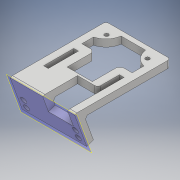
# Autodesk Inventor part: OpenMVMount-Tatev2
Saved by Autodesk Inventor 2018.3 (Build 223284000, 284)
## iProperties
Created: 2019-04-14
Part Number: OpenMVMount-Tatev2
Material: 一般
Document SubType Name: Modeling
Designer: shun2
Density: 1 g/cm^3
Appearance: 既定
Author: shun2
Autodesk Inventor part; units mm, degrees
(part 1 of 6)
ref_plane "YZ Plane" through (0, 0, 0) normal (1, 0, 0) x (0, 1, 0)
ref_plane "XZ Plane" through (0, 0, 0) normal (0, 1, 0) x (-1, 0, 0)
ref_plane "XY Plane" through (0, 0, 0) normal (0, 0, 1) x (1, 0, 0)
sketch "スケッチ1" plane through (0, 0, 0) normal (0, 0, 1) x (1, 0, 0)
  line L0 (0, 44.45) -> (0, 0)
  line L1 (0, 0) -> (35.56, 0)
  line L2 (35.56, 0) -> (35.56, 44.45)
  line L3 (35.56, 44.45) -> (0, 44.45)
  line L4 (3.8608, 3.6322) -> (3.1998, 3.6322)
  line L5 (3.1998, 3.6322) -> (3.1998, 3.9627)
  line L6 (3.1998, 3.9627) -> (3.31, 4.0728)
  line L7 (3.31, 4.0728) -> (3.5303, 4.0728)
  line L8 (3.5303, 4.0728) -> (3.6405, 3.9627)
  line L9 (3.6405, 3.9627) -> (3.6405, 3.6322)
  line L10 (3.1998, 4.8213) -> (3.31, 4.6009)
  line L11 (3.31, 4.6009) -> (3.5303, 4.3806)
  line L12 (3.5303, 4.3806) -> (3.7506, 4.3806)
  line L13 (3.7506, 4.3806) -> (3.8608, 4.4908)
  line L14 (3.8608, 4.4908) -> (3.8608, 4.7111)
  line L15 (3.8608, 4.7111) -> (3.7506, 4.8213)
  line L16 (3.7506, 4.8213) -> (3.6405, 4.8213)
  line L17 (3.6405, 4.8213) -> (3.5303, 4.7111)
  line L18 (3.5303, 4.7111) -> (3.5303, 4.3806)
  line L19 (3.8608, 8.5852) -> (3.1998, 8.5852)
  line L20 (3.1998, 8.5852) -> (3.1998, 8.9157)
  line L21 (3.1998, 8.9157) -> (3.31, 9.0258)
  line L22 (3.31, 9.0258) -> (3.5303, 9.0258)
  line L23 (3.5303, 9.0258) -> (3.6405, 8.9157)
  line L24 (3.6405, 8.9157) -> (3.6405, 8.5852)
  line L25 (3.8608, 9.6641) -> (3.1998, 9.6641)
  line L26 (3.1998, 9.6641) -> (3.5303, 9.3336)
  line L27 (3.5303, 9.3336) -> (3.5303, 9.7743)
  line L28 (3.8608, 6.0452) -> (3.1998, 6.0452)
  line L29 (3.1998, 6.0452) -> (3.1998, 6.3757)
  line L30 (3.1998, 6.3757) -> (3.31, 6.4858)
  line L31 (3.31, 6.4858) -> (3.5303, 6.4858)
  line L32 (3.5303, 6.4858) -> (3.6405, 6.3757)
  line L33 (3.6405, 6.3757) -> (3.6405, 6.0452)
  line L34 (3.1998, 7.2343) -> (3.1998, 6.7936)
  line L35 (3.1998, 6.7936) -> (3.5303, 6.7936)
  line L36 (3.5303, 6.7936) -> (3.4202, 7.0139)
  line L37 (3.4202, 7.0139) -> (3.4202, 7.1241)
  line L38 (3.4202, 7.1241) -> (3.5303, 7.2343)
  line L39 (3.5303, 7.2343) -> (3.7506, 7.2343)
  line L40 (3.7506, 7.2343) -> (3.8608, 7.1241)
  line L41 (3.8608, 7.1241) -> (3.8608, 6.9038)
  line L42 (3.8608, 6.9038) -> (3.7506, 6.7936)
  line L43 (3.8608, 11.1252) -> (3.1998, 11.1252)
  line L44 (3.1998, 11.1252) -> (3.1998, 11.4557)
  line L45 (3.1998, 11.4557) -> (3.31, 11.5658)
  line L46 (3.31, 11.5658) -> (3.5303, 11.5658)
  line L47 (3.5303, 11.5658) -> (3.6405, 11.4557)
  line L48 (3.6405, 11.4557) -> (3.6405, 11.1252)
  line L49 (3.31, 11.8736) -> (3.1998, 11.9838)
  line L50 (3.1998, 11.9838) -> (3.1998, 12.2041)
  line L51 (3.1998, 12.2041) -> (3.31, 12.3143)
  line L52 (3.31, 12.3143) -> (3.4202, 12.3143)
  line L53 (3.4202, 12.3143) -> (3.5303, 12.2041)
  line L54 (3.5303, 12.2041) -> (3.5303, 12.0939)
  line L55 (3.5303, 12.2041) -> (3.6405, 12.3143)
  line L56 (3.6405, 12.3143) -> (3.7506, 12.3143)
  line L57 (3.7506, 12.3143) -> (3.8608, 12.2041)
  line L58 (3.8608, 12.2041) -> (3.8608, 11.9838)
  line L59 (3.8608, 11.9838) -> (3.7506, 11.8736)
  line L60 (3.8608, 13.7922) -> (3.1998, 13.7922)
  line L61 (3.1998, 13.7922) -> (3.1998, 14.1227)
  line L62 (3.1998, 14.1227) -> (3.31, 14.2328)
  line L63 (3.31, 14.2328) -> (3.5303, 14.2328)
  line L64 (3.5303, 14.2328) -> (3.6405, 14.1227)
  line L65 (3.6405, 14.1227) -> (3.6405, 13.7922)
  line L66 (3.8608, 14.9813) -> (3.8608, 14.5406)
  line L67 (3.8608, 14.5406) -> (3.4202, 14.9813)
  line L68 (3.4202, 14.9813) -> (3.31, 14.9813)
  line L69 (3.31, 14.9813) -> (3.1998, 14.8711)
  line L70 (3.1998, 14.8711) -> (3.1998, 14.6508)
  line L71 (3.1998, 14.6508) -> (3.31, 14.5406)
  line L72 (3.8608, 16.3322) -> (3.1998, 16.3322)
  line L73 (3.1998, 16.3322) -> (3.1998, 16.6627)
  line L74 (3.1998, 16.6627) -> (3.31, 16.7728)
  line L75 (3.31, 16.7728) -> (3.5303, 16.7728)
  line L76 (3.5303, 16.7728) -> (3.6405, 16.6627)
  line L77 (3.6405, 16.6627) -> (3.6405, 16.3322)
  line L78 (3.4202, 17.0806) -> (3.1998, 17.3009)
  line L79 (3.1998, 17.3009) -> (3.8608, 17.3009)
  line L80 (3.8608, 17.0806) -> (3.8608, 17.5213)
  line L81 (27.821, 13.7248) -> (27.7108, 13.6147)
  line L82 (27.7108, 13.6147) -> (27.7108, 13.3944)
  line L83 (27.7108, 13.3944) -> (27.821, 13.2842)
  line L84 (27.821, 13.2842) -> (27.9312, 13.2842)
  line L85 (27.9312, 13.2842) -> (28.0413, 13.3944)
  line L86 (28.0413, 13.3944) -> (28.0413, 13.6147)
  line L87 (28.0413, 13.6147) -> (28.1515, 13.7248)
  line L88 (28.1515, 13.7248) -> (28.2616, 13.7248)
  line L89 (28.2616, 13.7248) -> (28.3718, 13.6147)
  line L90 (28.3718, 13.6147) -> (28.3718, 13.3944)
  line L91 (28.3718, 13.3944) -> (28.2616, 13.2842)
  line L92 (27.7108, 14.0326) -> (28.3718, 14.0326)
  line L93 (28.3718, 14.0326) -> (28.1515, 14.2529)
  line L94 (28.1515, 14.2529) -> (28.3718, 14.4733)
  line L95 (28.3718, 14.4733) -> (27.7108, 14.4733)
  line L96 (27.7108, 14.781) -> (28.3718, 14.781)
  line L97 (28.3718, 14.781) -> (28.3718, 15.1115)
  line L98 (28.3718, 15.1115) -> (28.2616, 15.2217)
  line L99 (28.2616, 15.2217) -> (27.821, 15.2217)
  line L100 (27.821, 15.2217) -> (27.7108, 15.1115)
  line L101 (27.7108, 15.1115) -> (27.7108, 14.781)
  line L102 (27.821, 16.2648) -> (27.7108, 16.1547)
  line L103 (27.7108, 16.1547) -> (27.7108, 15.9344)
  line L104 (27.7108, 15.9344) -> (27.821, 15.8242)
  line L105 (27.821, 15.8242) -> (27.9312, 15.8242)
  line L106 (27.9312, 15.8242) -> (28.0413, 15.9344)
  line L107 (28.0413, 15.9344) -> (28.0413, 16.1547)
  line L108 (28.0413, 16.1547) -> (28.1515, 16.2648)
  line L109 (28.1515, 16.2648) -> (28.2616, 16.2648)
  line L110 (28.2616, 16.2648) -> (28.3718, 16.1547)
  line L111 (28.3718, 16.1547) -> (28.3718, 15.9344)
  line L112 (28.3718, 15.9344) -> (28.2616, 15.8242)
  line L113 (27.7108, 16.5726) -> (28.3718, 16.5726)
  line L114 (28.3718, 16.5726) -> (28.1515, 16.7929)
  line L115 (28.1515, 16.7929) -> (28.3718, 17.0133)
  line L116 (28.3718, 17.0133) -> (27.7108, 17.0133)
  line L117 (27.821, 17.7617) -> (27.7108, 17.6515)
  line L118 (27.7108, 17.6515) -> (27.7108, 17.4312)
  line L119 (27.7108, 17.4312) -> (27.821, 17.321)
  line L120 (27.821, 17.321) -> (28.2616, 17.321)
  line L121 (28.2616, 17.321) -> (28.3718, 17.4312)
  line L122 (28.3718, 17.4312) -> (28.3718, 17.6515)
  line L123 (28.3718, 17.6515) -> (28.2616, 17.7617)
  line L124 (32.3088, 15.5067) -> (31.6987, 15.5067)
  line L125 (31.6987, 15.5067) -> (31.6987, 15.8118)
  line L126 (31.6987, 15.8118) -> (31.8004, 15.9134)
  line L127 (31.8004, 15.9134) -> (31.9021, 15.9134)
  line L128 (31.9021, 15.9134) -> (32.0037, 15.8118)
  line L129 (32.0037, 15.8118) -> (32.1054, 15.9134)
  line L130 (32.1054, 15.9134) -> (32.2071, 15.9134)
  line L131 (32.2071, 15.9134) -> (32.3088, 15.8118)
  line L132 (32.3088, 15.8118) -> (32.3088, 15.5067)
  line L133 (32.0037, 15.5067) -> (32.0037, 15.8118)
  line L134 (31.6987, 16.5134) -> (31.6987, 16.31)
  line L135 (31.6987, 16.31) -> (31.8004, 16.2083)
  line L136 (31.8004, 16.2083) -> (32.2071, 16.2083)
  line L137 (32.2071, 16.2083) -> (32.3088, 16.31)
  line L138 (32.3088, 16.31) -> (32.3088, 16.5134)
  line L139 (32.3088, 16.5134) -> (32.2071, 16.6151)
  line L140 (32.2071, 16.6151) -> (31.8004, 16.6151)
  line L141 (31.8004, 16.6151) -> (31.6987, 16.5134)
  line L142 (31.6987, 17.215) -> (31.6987, 17.0117)
  line L143 (31.6987, 17.0117) -> (31.8004, 16.91)
  line L144 (31.8004, 16.91) -> (32.2071, 16.91)
  line L145 (32.2071, 16.91) -> (32.3088, 17.0117)
  line L146 (32.3088, 17.0117) -> (32.3088, 17.215)
  line L147 (32.3088, 17.215) -> (32.2071, 17.3167)
  line L148 (32.2071, 17.3167) -> (31.8004, 17.3167)
  line L149 (31.8004, 17.3167) -> (31.6987, 17.215)
  line L150 (32.3088, 17.815) -> (31.6987, 17.815)
  line L151 (31.6987, 17.6116) -> (31.6987, 18.0184)
  line L152 (32.3088, 18.4912) -> (31.6478, 18.4912)
  line L153 (31.6478, 18.4912) -> (31.6478, 18.8217)
  line L154 (31.6478, 18.8217) -> (31.758, 18.9318)
  line L155 (31.758, 18.9318) -> (31.9783, 18.9318)
  line L156 (31.9783, 18.9318) -> (32.0885, 18.8217)
  line L157 (32.0885, 18.8217) -> (32.0885, 18.4912)
  line L158 (32.0885, 18.7115) -> (32.3088, 18.9318)
  line L159 (31.758, 19.6803) -> (31.6478, 19.5701)
  line L160 (31.6478, 19.5701) -> (31.6478, 19.3498)
  line L161 (31.6478, 19.3498) -> (31.758, 19.2396)
  line L162 (31.758, 19.2396) -> (31.8682, 19.2396)
  line L163 (31.8682, 19.2396) -> (31.9783, 19.3498)
  line L164 (31.9783, 19.3498) -> (31.9783, 19.5701)
  line L165 (31.9783, 19.5701) -> (32.0885, 19.6803)
  line L166 (32.0885, 19.6803) -> (32.1986, 19.6803)
  line L167 (32.1986, 19.6803) -> (32.3088, 19.5701)
  line L168 (32.3088, 19.5701) -> (32.3088, 19.3498)
  line L169 (32.3088, 19.3498) -> (32.1986, 19.2396)
  line L170 (32.3088, 20.2083) -> (31.6478, 20.2083)
  line L171 (31.6478, 19.988) -> (31.6478, 20.4287)
  line L172 (32.3088, 6.1722) -> (31.6478, 6.1722)
  line L173 (31.6478, 6.1722) -> (31.6478, 6.5027)
  line L174 (31.6478, 6.5027) -> (31.758, 6.6128)
  line L175 (31.758, 6.6128) -> (31.9783, 6.6128)
  line L176 (31.9783, 6.6128) -> (32.0885, 6.5027)
  line L177 (32.0885, 6.5027) -> (32.0885, 6.1722)
  line L178 (31.6478, 6.9206) -> (31.6478, 7.3613)
  line L179 (31.6478, 7.3613) -> (31.758, 7.3613)
  line L180 (31.758, 7.3613) -> (32.1986, 6.9206)
  line L181 (32.1986, 6.9206) -> (32.3088, 6.9206)
  line L182 (31.758, 1.1518) -> (31.6478, 1.0417)
  line L183 (31.6478, 1.0417) -> (31.6478, 0.8214)
  line L184 (31.6478, 0.8214) -> (31.758, 0.7112)
  line L185 (31.758, 0.7112) -> (32.1986, 0.7112)
  line L186 (32.1986, 0.7112) -> (32.3088, 0.8214)
  line L187 (32.3088, 0.8214) -> (32.3088, 1.0417)
  line L188 (32.3088, 1.0417) -> (32.1986, 1.1518)
  line L189 (32.1986, 1.1518) -> (31.9783, 1.1518)
  line L190 (31.9783, 1.1518) -> (31.9783, 0.9315)
  line L191 (32.3088, 1.4596) -> (31.6478, 1.4596)
  line L192 (31.6478, 1.4596) -> (32.3088, 1.9003)
  line L193 (32.3088, 1.9003) -> (31.6478, 1.9003)
  line L194 (31.6478, 2.208) -> (32.3088, 2.208)
  line L195 (32.3088, 2.208) -> (32.3088, 2.5385)
  line L196 (32.3088, 2.5385) -> (32.1986, 2.6487)
  line L197 (32.1986, 2.6487) -> (31.758, 2.6487)
  line L198 (31.758, 2.6487) -> (31.6478, 2.5385)
  line L199 (31.6478, 2.5385) -> (31.6478, 2.208)
  line L200 (3.31, 0.5842) -> (3.1998, 0.6944)
  line L201 (3.1998, 0.6944) -> (3.1998, 0.9147)
  line L202 (3.1998, 0.9147) -> (3.31, 1.0248)
  line L203 (3.31, 1.0248) -> (3.4202, 1.0248)
  line L204 (3.4202, 1.0248) -> (3.5303, 0.9147)
  line L205 (3.5303, 0.9147) -> (3.5303, 0.8045)
  line L206 (3.5303, 0.9147) -> (3.6405, 1.0248)
  line L207 (3.6405, 1.0248) -> (3.7506, 1.0248)
  line L208 (3.7506, 1.0248) -> (3.8608, 0.9147)
  line L209 (3.8608, 0.9147) -> (3.8608, 0.6944)
  line L210 (3.8608, 0.6944) -> (3.7506, 0.5842)
  line L211 (3.8608, 1.3326) -> (3.7506, 1.3326)
  line L212 (3.7506, 1.3326) -> (3.7506, 1.4428)
  line L213 (3.7506, 1.4428) -> (3.8608, 1.4428)
  line L214 (3.8608, 1.4428) -> (3.8608, 1.3326)
  line L215 (3.31, 1.7068) -> (3.1998, 1.817)
  line L216 (3.1998, 1.817) -> (3.1998, 2.0373)
  line L217 (3.1998, 2.0373) -> (3.31, 2.1475)
  line L218 (3.31, 2.1475) -> (3.4202, 2.1475)
  line L219 (3.4202, 2.1475) -> (3.5303, 2.0373)
  line L220 (3.5303, 2.0373) -> (3.5303, 1.9271)
  line L221 (3.5303, 2.0373) -> (3.6405, 2.1475)
  line L222 (3.6405, 2.1475) -> (3.7506, 2.1475)
  line L223 (3.7506, 2.1475) -> (3.8608, 2.0373)
  line L224 (3.8608, 2.0373) -> (3.8608, 1.817)
  line L225 (3.8608, 1.817) -> (3.7506, 1.7068)
  line L226 (3.1998, 2.4552) -> (3.6405, 2.4552)
  line L227 (3.6405, 2.4552) -> (3.8608, 2.6756)
  line L228 (3.8608, 2.6756) -> (3.6405, 2.8959)
  line L229 (3.6405, 2.8959) -> (3.1998, 2.8959)
  line L230 (31.6478, 3.2512) -> (32.0885, 3.2512)
  line L231 (32.0885, 3.2512) -> (32.3088, 3.4715)
  line L232 (32.3088, 3.4715) -> (32.0885, 3.6918)
  line L233 (32.0885, 3.6918) -> (31.6478, 3.6918)
  line L234 (32.3088, 3.9996) -> (32.3088, 4.2199)
  line L235 (32.3088, 4.1098) -> (31.6478, 4.1098)
  line L236 (31.6478, 3.9996) -> (31.6478, 4.2199)
  line L237 (32.3088, 4.4986) -> (31.6478, 4.4986)
  line L238 (31.6478, 4.4986) -> (32.3088, 4.9392)
  line L239 (32.3088, 4.9392) -> (31.6478, 4.9392)
  line L240 (32.3088, 8.5852) -> (31.6478, 8.5852)
  line L241 (31.6478, 8.5852) -> (31.6478, 8.9157)
  line L242 (31.6478, 8.9157) -> (31.758, 9.0258)
  line L243 (31.758, 9.0258) -> (31.9783, 9.0258)
  line L244 (31.9783, 9.0258) -> (32.0885, 8.9157)
  line L245 (32.0885, 8.9157) -> (32.0885, 8.5852)
  line L246 (31.758, 9.3336) -> (31.6478, 9.4438)
  line L247 (31.6478, 9.4438) -> (31.6478, 9.6641)
  line L248 (31.6478, 9.6641) -> (31.758, 9.7743)
  line L249 (31.758, 9.7743) -> (31.8682, 9.7743)
  line L250 (31.8682, 9.7743) -> (31.9783, 9.6641)
  line L251 (31.9783, 9.6641) -> (32.0885, 9.7743)
  line L252 (32.0885, 9.7743) -> (32.1986, 9.7743)
  line L253 (32.1986, 9.7743) -> (32.3088, 9.6641)
  line L254 (32.3088, 9.6641) -> (32.3088, 9.4438)
  line L255 (32.3088, 9.4438) -> (32.1986, 9.3336)
  line L256 (32.1986, 9.3336) -> (32.0885, 9.3336)
  line L257 (32.0885, 9.3336) -> (31.9783, 9.4438)
  line L258 (31.9783, 9.4438) -> (31.8682, 9.3336)
  line L259 (31.8682, 9.3336) -> (31.758, 9.3336)
  line L260 (31.9783, 9.4438) -> (31.9783, 9.6641)
  line L261 (3.8608, 18.8722) -> (3.1998, 18.8722)
  line L262 (3.1998, 18.8722) -> (3.1998, 19.2027)
  line L263 (3.1998, 19.2027) -> (3.31, 19.3128)
  line L264 (3.31, 19.3128) -> (3.5303, 19.3128)
  line L265 (3.5303, 19.3128) -> (3.6405, 19.2027)
  line L266 (3.6405, 19.2027) -> (3.6405, 18.8722)
  line L267 (3.7506, 19.6206) -> (3.31, 19.6206)
  line L268 (3.31, 19.6206) -> (3.1998, 19.7308)
  line L269 (3.1998, 19.7308) -> (3.1998, 19.9511)
  line L270 (3.1998, 19.9511) -> (3.31, 20.0613)
  line L271 (3.31, 20.0613) -> (3.7506, 20.0613)
  line L272 (3.7506, 20.0613) -> (3.8608, 19.9511)
  line L273 (3.8608, 19.9511) -> (3.8608, 19.7308)
  line L274 (3.8608, 19.7308) -> (3.7506, 19.6206)
  line L275 (3.7506, 19.6206) -> (3.31, 20.0613)
  line L276 (28.3718, 10.8712) -> (27.7108, 10.8712)
  line L277 (27.7108, 10.8712) -> (27.7108, 11.2017)
  line L278 (27.7108, 11.2017) -> (27.821, 11.3118)
  line L279 (27.821, 11.3118) -> (28.0413, 11.3118)
  line L280 (28.0413, 11.3118) -> (28.1515, 11.2017)
  line L281 (28.1515, 11.2017) -> (28.1515, 10.8712)
  line L282 (28.1515, 11.0915) -> (28.3718, 11.3118)
  line L283 (27.821, 12.0603) -> (27.7108, 11.9501)
  line L284 (27.7108, 11.9501) -> (27.7108, 11.7298)
  line L285 (27.7108, 11.7298) -> (27.821, 11.6196)
  line L286 (27.821, 11.6196) -> (27.9312, 11.6196)
  line L287 (27.9312, 11.6196) -> (28.0413, 11.7298)
  line L288 (28.0413, 11.7298) -> (28.0413, 11.9501)
  line L289 (28.0413, 11.9501) -> (28.1515, 12.0603)
  line L290 (28.1515, 12.0603) -> (28.2616, 12.0603)
  line L291 (28.2616, 12.0603) -> (28.3718, 11.9501)
  line L292 (28.3718, 11.9501) -> (28.3718, 11.7298)
  line L293 (28.3718, 11.7298) -> (28.2616, 11.6196)
  line L294 (28.3718, 12.5884) -> (27.7108, 12.5884)
  line L295 (27.7108, 12.368) -> (27.7108, 12.8087)
  line L296 (27.821, 6.1048) -> (27.7108, 5.9947)
  line L297 (27.7108, 5.9947) -> (27.7108, 5.7744)
  line L298 (27.7108, 5.7744) -> (27.821, 5.6642)
  line L299 (27.821, 5.6642) -> (28.2616, 5.6642)
  line L300 (28.2616, 5.6642) -> (28.3718, 5.7744)
  line L301 (28.3718, 5.7744) -> (28.3718, 5.9947)
  line L302 (28.3718, 5.9947) -> (28.2616, 6.1048)
  line L303 (28.2616, 6.1048) -> (28.0413, 6.1048)
  line L304 (28.0413, 6.1048) -> (28.0413, 5.8845)
  line L305 (28.3718, 6.4126) -> (27.7108, 6.4126)
  line L306 (27.7108, 6.4126) -> (28.3718, 6.8533)
  line L307 (28.3718, 6.8533) -> (27.7108, 6.8533)
  line L308 (27.7108, 7.161) -> (28.3718, 7.161)
  line L309 (28.3718, 7.161) -> (28.3718, 7.4915)
  line L310 (28.3718, 7.4915) -> (28.2616, 7.6017)
  line L311 (28.2616, 7.6017) -> (27.821, 7.6017)
  line L312 (27.821, 7.6017) -> (27.7108, 7.4915)
  line L313 (27.7108, 7.4915) -> (27.7108, 7.161)
  line L314 (27.821, 8.0772) -> (27.7108, 8.1874)
  line L315 (27.7108, 8.1874) -> (27.7108, 8.4077)
  line L316 (27.7108, 8.4077) -> (27.821, 8.5178)
  line L317 (27.821, 8.5178) -> (27.9312, 8.5178)
  line L318 (27.9312, 8.5178) -> (28.0413, 8.4077)
  line L319 (28.0413, 8.4077) -> (28.0413, 8.2975)
  line L320 (28.0413, 8.4077) -> (28.1515, 8.5178)
  line L321 (28.1515, 8.5178) -> (28.2616, 8.5178)
  line L322 (28.2616, 8.5178) -> (28.3718, 8.4077)
  line L323 (28.3718, 8.4077) -> (28.3718, 8.1874)
  line L324 (28.3718, 8.1874) -> (28.2616, 8.0772)
  line L325 (28.3718, 8.8256) -> (28.2616, 8.8256)
  line L326 (28.2616, 8.8256) -> (28.2616, 8.9358)
  line L327 (28.2616, 8.9358) -> (28.3718, 8.9358)
  line L328 (28.3718, 8.9358) -> (28.3718, 8.8256)
  line L329 (27.821, 9.1998) -> (27.7108, 9.31)
  line L330 (27.7108, 9.31) -> (27.7108, 9.5303)
  line L331 (27.7108, 9.5303) -> (27.821, 9.6405)
  line L332 (27.821, 9.6405) -> (27.9312, 9.6405)
  line L333 (27.9312, 9.6405) -> (28.0413, 9.5303)
  line L334 (28.0413, 9.5303) -> (28.0413, 9.4201)
  line L335 (28.0413, 9.5303) -> (28.1515, 9.6405)
  line L336 (28.1515, 9.6405) -> (28.2616, 9.6405)
  line L337 (28.2616, 9.6405) -> (28.3718, 9.5303)
  line L338 (28.3718, 9.5303) -> (28.3718, 9.31)
  line L339 (28.3718, 9.31) -> (28.2616, 9.1998)
  line L340 (27.9312, 9.9482) -> (28.3718, 10.1686)
  line L341 (28.3718, 10.1686) -> (27.9312, 10.3889)
  line L342 (31.758, 13.4708) -> (31.6478, 13.3607)
  line L343 (31.6478, 13.3607) -> (31.6478, 13.1404)
  line L344 (31.6478, 13.1404) -> (31.758, 13.0302)
  line L345 (31.758, 13.0302) -> (31.8682, 13.0302)
  line L346 (31.8682, 13.0302) -> (31.9783, 13.1404)
  line L347 (31.9783, 13.1404) -> (31.9783, 13.3607)
  line L348 (31.9783, 13.3607) -> (32.0885, 13.4708)
  line L349 (32.0885, 13.4708) -> (32.1986, 13.4708)
  line L350 (32.1986, 13.4708) -> (32.3088, 13.3607)
  line L351 (32.3088, 13.3607) -> (32.3088, 13.1404)
  line L352 (32.3088, 13.1404) -> (32.1986, 13.0302)
  line L353 (31.6478, 13.7786) -> (31.758, 13.7786)
  line L354 (31.758, 13.7786) -> (31.9783, 13.9989)
  line L355 (31.9783, 13.9989) -> (31.758, 14.2193)
  line L356 (31.758, 14.2193) -> (31.6478, 14.2193)
  line L357 (31.9783, 13.9989) -> (32.3088, 13.9989)
  line L358 (32.3088, 14.527) -> (31.6478, 14.527)
  line L359 (31.6478, 14.527) -> (32.3088, 14.9677)
  line L360 (32.3088, 14.9677) -> (31.6478, 14.9677)
  line L361 (32.3088, 11.1252) -> (31.6478, 11.1252)
  line L362 (31.6478, 11.1252) -> (31.6478, 11.4557)
  line L363 (31.6478, 11.4557) -> (31.758, 11.5658)
  line L364 (31.758, 11.5658) -> (31.9783, 11.5658)
  line L365 (31.9783, 11.5658) -> (32.0885, 11.4557)
  line L366 (32.0885, 11.4557) -> (32.0885, 11.1252)
  line L367 (32.1986, 11.8736) -> (32.3088, 11.9838)
  line L368 (32.3088, 11.9838) -> (32.3088, 12.2041)
  line L369 (32.3088, 12.2041) -> (32.1986, 12.3143)
  line L370 (32.1986, 12.3143) -> (31.758, 12.3143)
  line L371 (31.758, 12.3143) -> (31.6478, 12.2041)
  line L372 (31.6478, 12.2041) -> (31.6478, 11.9838)
  line L373 (31.6478, 11.9838) -> (31.758, 11.8736)
  line L374 (31.758, 11.8736) -> (31.8682, 11.8736)
  line L375 (31.8682, 11.8736) -> (31.9783, 11.9838)
  line L376 (31.9783, 11.9838) -> (31.9783, 12.3143)
  line L377 (27.878, 25.397) -> (26.478, 25.397)
  line L378 (26.478, 25.397) -> (26.478, 28.197)
  line L379 (26.478, 28.197) -> (27.878, 28.197)
  line L380 (27.878, 28.197) -> (27.878, 25.397)
  line L381 (17.21, 1.902) -> (15.81, 1.902)
  line L382 (15.81, 1.902) -> (15.81, 4.702)
  line L383 (15.81, 4.702) -> (17.21, 4.702)
  line L384 (17.21, 4.702) -> (17.21, 1.902)
  line L385 (7.423, 1.921) -> (7.423, 0.421)
  line L386 (7.423, 0.421) -> (5.023, 0.421)
  line L387 (5.023, 0.421) -> (5.023, 1.921)
  line L388 (7.423, 3.921) -> (7.423, 5.021)
  line L389 (7.423, 5.021) -> (7.023, 5.421)
  line L390 (7.023, 5.421) -> (5.423, 5.421)
  line L391 (5.423, 5.421) -> (5.023, 5.021)
  line L392 (5.023, 5.021) -> (5.023, 3.921)
  line L393 (5.207, 3.302) -> (7.239, 3.302)
  line L394 (8.2855, 10.414) -> (8.2245, 10.414)
  line L395 (8.955, 11.914) -> (8.955, 8.914)
  line L396 (8.955, 8.914) -> (7.555, 8.914)
  line L397 (7.555, 8.914) -> (7.555, 11.914)
  line L398 (7.555, 11.914) -> (8.955, 11.914)
  line L399 (6.6345, 10.414) -> (6.5735, 10.414)
  line L400 (7.304, 11.914) -> (7.304, 8.914)
  line L401 (7.304, 8.914) -> (5.904, 8.914)
  line L402 (5.904, 8.914) -> (5.904, 11.914)
  line L403 (5.904, 11.914) -> (7.304, 11.914)
  line L404 (10.1295, 25.019) -> (10.1905, 25.019)
  line L405 (9.46, 23.519) -> (9.46, 26.519)
  line L406 (9.46, 26.519) -> (10.86, 26.519)
  line L407 (10.86, 26.519) -> (10.86, 23.519)
  line L408 (10.86, 23.519) -> (9.46, 23.519)
  line L409 (12.065, 6.4465) -> (12.065, 6.5075)
  line L410 (13.565, 5.777) -> (10.565, 5.777)
  line L411 (10.565, 5.777) -> (10.565, 7.177)
  line L412 (10.565, 7.177) -> (13.565, 7.177)
  line L413 (13.565, 7.177) -> (13.565, 5.777)
  line L414 (25.5575, 7.747) -> (25.4965, 7.747)
  line L415 (26.227, 9.247) -> (26.227, 6.247)
  line L416 (26.227, 6.247) -> (24.827, 6.247)
  line L417 (24.827, 6.247) -> (24.827, 9.247)
  line L418 (24.827, 9.247) -> (26.227, 9.247)
  line L419 (25.4965, 25.019) -> (25.5575, 25.019)
  line L420 (24.827, 23.519) -> (24.827, 26.519)
  line L421 (24.827, 26.519) -> (26.227, 26.519)
  line L422 (26.227, 26.519) -> (26.227, 23.519)
  line L423 (26.227, 23.519) -> (24.827, 23.519)
  line L424 (28.8595, 26.797) -> (28.7985, 26.797)
  line L425 (29.529, 28.297) -> (29.529, 25.297)
  line L426 (29.529, 25.297) -> (28.129, 25.297)
  line L427 (28.129, 25.297) -> (28.129, 28.297)
  line L428 (28.129, 28.297) -> (29.529, 28.297)
  line L429 (6.928, 26.273) -> (6.928, 27.773)
  line L430 (6.928, 27.773) -> (9.328, 27.773)
  line L431 (9.328, 27.773) -> (9.328, 26.273)
  line L432 (6.928, 24.273) -> (6.928, 23.173)
  line L433 (6.928, 23.173) -> (7.328, 22.773)
  line L434 (7.328, 22.773) -> (8.928, 22.773)
  line L435 (8.928, 22.773) -> (9.328, 23.173)
  line L436 (9.328, 23.173) -> (9.328, 24.273)
  line L437 (9.144, 24.892) -> (7.112, 24.892)
  line L438 (22.971, 41.967) -> (24.471, 41.967)
  line L439 (24.471, 41.967) -> (24.471, 39.567)
  line L440 (24.471, 39.567) -> (22.971, 39.567)
  line L441 (20.971, 41.967) -> (19.871, 41.967)
  line L442 (19.871, 41.967) -> (19.471, 41.567)
  line L443 (19.471, 41.567) -> (19.471, 39.967)
  line L444 (19.471, 39.967) -> (19.871, 39.567)
  line L445 (19.871, 39.567) -> (20.971, 39.567)
  line L446 (21.59, 39.751) -> (21.59, 41.783)
  line L447 (8.2245, 19.812) -> (8.2855, 19.812)
  line L448 (7.555, 18.312) -> (7.555, 21.312)
  line L449 (7.555, 21.312) -> (8.955, 21.312)
  line L450 (8.955, 21.312) -> (8.955, 18.312)
  line L451 (8.955, 18.312) -> (7.555, 18.312)
  line L452 (17.673, 40.4695) -> (17.673, 40.5305)
  line L453 (19.173, 39.8) -> (16.173, 39.8)
  line L454 (16.173, 39.8) -> (16.173, 41.2)
  line L455 (16.173, 41.2) -> (19.173, 41.2)
  line L456 (19.173, 41.2) -> (19.173, 39.8)
  line L457 (22.0305, 35.9) -> (21.9695, 35.9)
  line L458 (22.7, 37.4) -> (22.7, 34.4)
  line L459 (22.7, 34.4) -> (21.3, 34.4)
  line L460 (21.3, 34.4) -> (21.3, 37.4)
  line L461 (21.3, 37.4) -> (22.7, 37.4)
  line L462 (19.3, 32.0695) -> (19.3, 32.1305)
  line L463 (20.8, 31.4) -> (17.8, 31.4)
  line L464 (17.8, 31.4) -> (17.8, 32.8)
  line L465 (17.8, 32.8) -> (20.8, 32.8)
  line L466 (20.8, 32.8) -> (20.8, 31.4)
  line L467 (22.0305, 32.2) -> (21.9695, 32.2)
  line L468 (22.7, 33.7) -> (22.7, 30.7)
  line L469 (22.7, 30.7) -> (21.3, 30.7)
  line L470 (21.3, 30.7) -> (21.3, 33.7)
  line L471 (21.3, 33.7) -> (22.7, 33.7)
  line L472 (13.7305, 37.6) -> (13.6695, 37.6)
  line L473 (14.4, 39.1) -> (14.4, 36.1)
  line L474 (14.4, 36.1) -> (13, 36.1)
  line L475 (13, 36.1) -> (13, 39.1)
  line L476 (13, 39.1) -> (14.4, 39.1)
  line L477 (12.7, 36.2) -> (11.3, 36.2)
  line L478 (11.3, 36.2) -> (11.3, 39)
  line L479 (11.3, 39) -> (12.7, 39)
  line L480 (12.7, 39) -> (12.7, 36.2)
  line L481 (5.842, 14.0005) -> (5.842, 13.9395)
  line L482 (4.342, 14.67) -> (7.342, 14.67)
  line L483 (7.342, 14.67) -> (7.342, 13.27)
  line L484 (7.342, 13.27) -> (4.342, 13.27)
  line L485 (4.342, 13.27) -> (4.342, 14.67)
  line L486 (5.842, 19.5275) -> (5.842, 19.5885)
  line L487 (7.342, 18.858) -> (4.342, 18.858)
  line L488 (4.342, 18.858) -> (4.342, 20.258)
  line L489 (4.342, 20.258) -> (7.342, 20.258)
  line L490 (7.342, 20.258) -> (7.342, 18.858)
  line L491 (29.3586, 19.8336) -> (29.3154, 19.7904)
  line L492 (28.7713, 21.3676) -> (30.8926, 19.2463)
  line L493 (30.8926, 19.2463) -> (29.9027, 18.2564)
  line L494 (29.9027, 18.2564) -> (27.7814, 20.3777)
  line L495 (27.7814, 20.3777) -> (28.7713, 21.3676)
  line L496 (19.685, 6.4465) -> (19.685, 6.5075)
  line L497 (21.185, 5.777) -> (18.185, 5.777)
  line L498 (18.185, 5.777) -> (18.185, 7.177)
  line L499 (18.185, 7.177) -> (21.185, 7.177)
  line L500 (21.185, 7.177) -> (21.185, 5.777)
  line L501 (18.0086, 3.2766) -> (18.0086, 4.0894)
  line L502 (18.0086, 4.0894) -> (18.5674, 4.0894)
  line L503 (20.8534, 4.0894) -> (20.8534, 3.2766)
  line L504 (20.2946, 4.0894) -> (20.8534, 4.0894)
  line L505 (0.381, 41.148) -> (0.635, 41.148)
  line L506 (5.969, 41.148) -> (6.223, 41.148)
  circle A0 centre (3.302, 41.148) radius 2.921
  circle A1 centre (3.302, 41.148) radius 1.5
  line L507 (35.179, 41.148) -> (34.925, 41.148)
  line L508 (29.591, 41.148) -> (29.337, 41.148)
  circle A2 centre (32.258, 41.148) radius 2.921
  circle A3 centre (32.258, 41.148) radius 1.5
  line L509 (35.179, 4.699) -> (35.179, 3.429)
  line L510 (35.179, 3.429) -> (34.544, 2.794)
  line L511 (34.544, 2.794) -> (33.274, 2.794)
  line L512 (33.274, 2.794) -> (32.639, 3.429)
  line L513 (34.544, 7.874) -> (35.179, 7.239)
  line L514 (35.179, 7.239) -> (35.179, 5.969)
  line L515 (35.179, 5.969) -> (34.544, 5.334)
  line L516 (34.544, 5.334) -> (33.274, 5.334)
  line L517 (33.274, 5.334) -> (32.639, 5.969)
  line L518 (32.639, 5.969) -> (32.639, 7.239)
  line L519 (32.639, 7.239) -> (33.274, 7.874)
  line L520 (35.179, 4.699) -> (34.544, 5.334)
  line L521 (33.274, 5.334) -> (32.639, 4.699)
  line L522 (32.639, 3.429) -> (32.639, 4.699)
  line L523 (35.179, 12.319) -> (35.179, 11.049)
  line L524 (35.179, 11.049) -> (34.544, 10.414)
  line L525 (34.544, 10.414) -> (33.274, 10.414)
  line L526 (33.274, 10.414) -> (32.639, 11.049)
  line L527 (34.544, 10.414) -> (35.179, 9.779)
  line L528 (35.179, 9.779) -> (35.179, 8.509)
  line L529 (35.179, 8.509) -> (34.544, 7.874)
  line L530 (34.544, 7.874) -> (33.274, 7.874)
  line L531 (33.274, 7.874) -> (32.639, 8.509)
  line L532 (32.639, 8.509) -> (32.639, 9.779)
  line L533 (32.639, 9.779) -> (33.274, 10.414)
  line L534 (34.544, 15.494) -> (35.179, 14.859)
  line L535 (35.179, 14.859) -> (35.179, 13.589)
  line L536 (35.179, 13.589) -> (34.544, 12.954)
  line L537 (34.544, 12.954) -> (33.274, 12.954)
  line L538 (33.274, 12.954) -> (32.639, 13.589)
  line L539 (32.639, 13.589) -> (32.639, 14.859)
  line L540 (32.639, 14.859) -> (33.274, 15.494)
  line L541 (35.179, 12.319) -> (34.544, 12.954)
  line L542 (33.274, 12.954) -> (32.639, 12.319)
  line L543 (32.639, 11.049) -> (32.639, 12.319)
  line L544 (35.179, 19.939) -> (35.179, 18.669)
  line L545 (35.179, 18.669) -> (34.544, 18.034)
  line L546 (34.544, 18.034) -> (33.274, 18.034)
  line L547 (33.274, 18.034) -> (32.639, 18.669)
  line L548 (34.544, 18.034) -> (35.179, 17.399)
  line L549 (35.179, 17.399) -> (35.179, 16.129)
  line L550 (35.179, 16.129) -> (34.544, 15.494)
  line L551 (34.544, 15.494) -> (33.274, 15.494)
  line L552 (33.274, 15.494) -> (32.639, 16.129)
  line L553 (32.639, 16.129) -> (32.639, 17.399)
  line L554 (32.639, 17.399) -> (33.274, 18.034)
  line L555 (34.544, 20.574) -> (33.274, 20.574)
  line L556 (35.179, 19.939) -> (34.544, 20.574)
  line L557 (33.274, 20.574) -> (32.639, 19.939)
  line L558 (32.639, 18.669) -> (32.639, 19.939)
  line L559 (35.179, 2.159) -> (35.179, 0.889)
  line L560 (35.179, 0.889) -> (34.544, 0.254)
  line L561 (34.544, 0.254) -> (33.274, 0.254)
  line L562 (33.274, 0.254) -> (32.639, 0.889)
  line L563 (35.179, 2.159) -> (34.544, 2.794)
  line L564 (33.274, 2.794) -> (32.639, 2.159)
  line L565 (32.639, 0.889) -> (32.639, 2.159)
  line L566 (2.921, 4.699) -> (2.921, 3.429)
  line L567 (2.921, 3.429) -> (2.286, 2.794)
  line L568 (2.286, 2.794) -> (1.016, 2.794)
  line L569 (1.016, 2.794) -> (0.381, 3.429)
  line L570 (2.286, 7.874) -> (2.921, 7.239)
  line L571 (2.921, 7.239) -> (2.921, 5.969)
  line L572 (2.921, 5.969) -> (2.286, 5.334)
  line L573 (2.286, 5.334) -> (1.016, 5.334)
  line L574 (1.016, 5.334) -> (0.381, 5.969)
  line L575 (0.381, 5.969) -> (0.381, 7.239)
  line L576 (0.381, 7.239) -> (1.016, 7.874)
  line L577 (2.921, 4.699) -> (2.286, 5.334)
  line L578 (1.016, 5.334) -> (0.381, 4.699)
  line L579 (0.381, 3.429) -> (0.381, 4.699)
  line L580 (2.921, 12.319) -> (2.921, 11.049)
  line L581 (2.921, 11.049) -> (2.286, 10.414)
  line L582 (2.286, 10.414) -> (1.016, 10.414)
  line L583 (1.016, 10.414) -> (0.381, 11.049)
  line L584 (2.286, 10.414) -> (2.921, 9.779)
  line L585 (2.921, 9.779) -> (2.921, 8.509)
  line L586 (2.921, 8.509) -> (2.286, 7.874)
  line L587 (2.286, 7.874) -> (1.016, 7.874)
  line L588 (1.016, 7.874) -> (0.381, 8.509)
  line L589 (0.381, 8.509) -> (0.381, 9.779)
  line L590 (0.381, 9.779) -> (1.016, 10.414)
  line L591 (2.286, 15.494) -> (2.921, 14.859)
  line L592 (2.921, 14.859) -> (2.921, 13.589)
  line L593 (2.921, 13.589) -> (2.286, 12.954)
  line L594 (2.286, 12.954) -> (1.016, 12.954)
  line L595 (1.016, 12.954) -> (0.381, 13.589)
  line L596 (0.381, 13.589) -> (0.381, 14.859)
  line L597 (0.381, 14.859) -> (1.016, 15.494)
  line L598 (2.921, 12.319) -> (2.286, 12.954)
  line L599 (1.016, 12.954) -> (0.381, 12.319)
  line L600 (0.381, 11.049) -> (0.381, 12.319)
  line L601 (2.921, 19.939) -> (2.921, 18.669)
  line L602 (2.921, 18.669) -> (2.286, 18.034)
  line L603 (2.286, 18.034) -> (1.016, 18.034)
  line L604 (1.016, 18.034) -> (0.381, 18.669)
  line L605 (2.286, 18.034) -> (2.921, 17.399)
  line L606 (2.921, 17.399) -> (2.921, 16.129)
  line L607 (2.921, 16.129) -> (2.286, 15.494)
  line L608 (2.286, 15.494) -> (1.016, 15.494)
  line L609 (1.016, 15.494) -> (0.381, 16.129)
  line L610 (0.381, 16.129) -> (0.381, 17.399)
  line L611 (0.381, 17.399) -> (1.016, 18.034)
  line L612 (2.286, 20.574) -> (1.016, 20.574)
  line L613 (2.921, 19.939) -> (2.286, 20.574)
  line L614 (1.016, 20.574) -> (0.381, 19.939)
  line L615 (0.381, 18.669) -> (0.381, 19.939)
  line L616 (2.921, 2.159) -> (2.921, 0.889)
  line L617 (2.921, 0.889) -> (2.286, 0.254)
  line L618 (2.286, 0.254) -> (1.016, 0.254)
  line L619 (1.016, 0.254) -> (0.381, 0.889)
  line L620 (2.921, 2.159) -> (2.286, 2.794)
  line L621 (1.016, 2.794) -> (0.381, 2.159)
  line L622 (0.381, 0.889) -> (0.381, 2.159)
  line L623 (31.369, 9.779) -> (31.369, 8.509)
  line L624 (31.369, 8.509) -> (30.734, 7.874)
  line L625 (30.734, 7.874) -> (29.464, 7.874)
  line L626 (29.464, 7.874) -> (28.829, 8.509)
  line L627 (30.734, 12.954) -> (31.369, 12.319)
  line L628 (31.369, 12.319) -> (31.369, 11.049)
  line L629 (31.369, 11.049) -> (30.734, 10.414)
  line L630 (30.734, 10.414) -> (29.464, 10.414)
  line L631 (29.464, 10.414) -> (28.829, 11.049)
  line L632 (28.829, 11.049) -> (28.829, 12.319)
  line L633 (28.829, 12.319) -> (29.464, 12.954)
  line L634 (31.369, 9.779) -> (30.734, 10.414)
  line L635 (29.464, 10.414) -> (28.829, 9.779)
  line L636 (28.829, 8.509) -> (28.829, 9.779)
  line L637 (31.369, 17.399) -> (31.369, 16.129)
  line L638 (31.369, 16.129) -> (30.734, 15.494)
  line L639 (30.734, 15.494) -> (29.464, 15.494)
  line L640 (29.464, 15.494) -> (28.829, 16.129)
  line L641 (30.734, 15.494) -> (31.369, 14.859)
  line L642 (31.369, 14.859) -> (31.369, 13.589)
  line L643 (31.369, 13.589) -> (30.734, 12.954)
  line L644 (30.734, 12.954) -> (29.464, 12.954)
  line L645 (29.464, 12.954) -> (28.829, 13.589)
  line L646 (28.829, 13.589) -> (28.829, 14.859)
  line L647 (28.829, 14.859) -> (29.464, 15.494)
  line L648 (30.734, 18.034) -> (29.464, 18.034)
  line L649 (31.369, 17.399) -> (30.734, 18.034)
  line L650 (29.464, 18.034) -> (28.829, 17.399)
  line L651 (28.829, 16.129) -> (28.829, 17.399)
  line L652 (31.369, 7.239) -> (31.369, 5.969)
  line L653 (31.369, 5.969) -> (30.734, 5.334)
  line L654 (30.734, 5.334) -> (29.464, 5.334)
  line L655 (29.464, 5.334) -> (28.829, 5.969)
  line L656 (31.369, 7.239) -> (30.734, 7.874)
  line L657 (29.464, 7.874) -> (28.829, 7.239)
  line L658 (28.829, 5.969) -> (28.829, 7.239)
  line L659 (5.653, 11.914) -> (5.653, 8.914)
  line L660 (5.653, 8.914) -> (4.253, 8.914)
  line L661 (4.253, 8.914) -> (4.253, 11.914)
  line L662 (4.253, 11.914) -> (5.653, 11.914)
  line L663 (24.487, 5.777) -> (21.487, 5.777)
  line L664 (21.487, 5.777) -> (21.487, 7.177)
  line L665 (21.487, 7.177) -> (24.487, 7.177)
  line L666 (24.487, 7.177) -> (24.487, 5.777)
  line L667 (1.24, 31.399) -> (0.94, 31.399)
  line L668 (0.94, 31.399) -> (0.94, 28.799)
  line L669 (0.94, 28.799) -> (1.24, 28.799)
  line L670 (3.84, 31.399) -> (4.14, 31.399)
  line L671 (4.14, 31.399) -> (4.14, 28.799)
  line L672 (4.14, 28.799) -> (3.84, 28.799)
  line L673 (3.94, 31.899) -> (3.94, 32.499)
  line L674 (3.94, 32.499) -> (3.34, 32.499)
  line L675 (33.1614, 34.4142) -> (33.5857, 33.9899)
  line L676 (33.5857, 33.9899) -> (34.7171, 35.1213)
  line L677 (34.7171, 35.1213) -> (34.2928, 35.5456)
  line L678 (31.7472, 35.8284) -> (31.3229, 36.2527)
  line L679 (31.3229, 36.2527) -> (32.4543, 37.3841)
  line L680 (32.4543, 37.3841) -> (32.8786, 36.9598)
  line L681 (32.3129, 35.4042) -> (32.8079, 35.8991)
  line L682 (32.8079, 35.8991) -> (33.3028, 36.3941)
  line L683 (32.8079, 35.8991) -> (32.8079, 35.0506)
  line L684 (32.8079, 35.0506) -> (33.6564, 35.8991)
  line L685 (33.6564, 35.8991) -> (32.8079, 35.8991)
  line L686 (3.8128, 35.8284) -> (4.2371, 36.2527)
  line L687 (4.2371, 36.2527) -> (3.1057, 37.3841)
  line L688 (3.1057, 37.3841) -> (2.6814, 36.9598)
  line L689 (2.3986, 34.4142) -> (1.9743, 33.9899)
  line L690 (1.9743, 33.9899) -> (0.8429, 35.1213)
  line L691 (0.8429, 35.1213) -> (1.2672, 35.5456)
  line L692 (2.8228, 34.9799) -> (2.3279, 35.4749)
  line L693 (2.3279, 35.4749) -> (1.8329, 35.9698)
  line L694 (2.3279, 35.4749) -> (3.1764, 35.4749)
  line L695 (3.1764, 35.4749) -> (2.3279, 36.3234)
  line L696 (2.3279, 36.3234) -> (2.3279, 35.4749)
  line L697 (9.78, 28.068) -> (9.78, 34.091)
  line L698 (9.78, 34.091) -> (9.78, 38.045)
  line L699 (9.78, 38.045) -> (9.78, 44.068)
  line L700 (9.78, 44.068) -> (25.78, 44.068)
  line L701 (25.78, 44.068) -> (25.78, 38.045)
  line L702 (25.78, 38.045) -> (25.78, 34.091)
  line L703 (25.78, 34.091) -> (25.78, 28.068)
  line L704 (25.78, 28.068) -> (9.78, 28.068)
  arc A4 (9.78, 38.045) -> (9.78, 34.091) centre (7.803, 36.068) ccw
  arc A5 (25.78, 34.091) -> (25.78, 38.045) centre (27.757, 36.068) ccw
  line L705 (10.78, 29.068) -> (24.78, 29.068)
  line L706 (24.78, 29.068) -> (24.78, 43.068)
  line L707 (24.78, 43.068) -> (10.78, 43.068)
  line L708 (10.78, 43.068) -> (10.78, 29.068)
  line L709 (27.051, 40.005) -> (26.67, 39.878)
  line L710 (26.67, 39.878) -> (26.543, 40.005)
  line L711 (26.543, 40.005) -> (26.797, 40.386)
  line L712 (26.797, 40.386) -> (26.543, 40.767)
  line L713 (26.543, 40.767) -> (26.289, 40.767)
  line L714 (26.289, 40.767) -> (26.289, 41.021)
  line L715 (26.289, 41.021) -> (26.67, 41.021)
  line L716 (26.67, 41.021) -> (26.797, 41.402)
  line L717 (26.797, 41.402) -> (26.543, 41.783)
  line L718 (26.543, 41.783) -> (26.67, 41.91)
  line L719 (26.67, 41.91) -> (27.051, 41.656)
  line L720 (27.051, 41.656) -> (27.432, 41.91)
  line L721 (27.432, 41.91) -> (27.432, 42.164)
  line L722 (27.432, 42.164) -> (27.686, 42.164)
  line L723 (27.686, 42.164) -> (27.813, 41.783)
  line L724 (27.813, 41.783) -> (28.194, 41.656)
  line L725 (28.194, 41.656) -> (28.448, 41.91)
  line L726 (28.448, 41.91) -> (28.575, 41.783)
  line L727 (28.575, 41.783) -> (28.448, 41.402)
  line L728 (28.448, 41.402) -> (28.575, 41.021)
  line L729 (28.575, 41.021) -> (28.956, 41.021)
  line L730 (28.956, 41.021) -> (28.829, 40.767)
  line L731 (28.829, 40.767) -> (28.448, 40.64)
  line L732 (28.448, 40.64) -> (28.448, 40.259)
  line L733 (28.448, 40.259) -> (28.575, 40.005)
  line L734 (28.575, 40.005) -> (28.448, 39.878)
  line L735 (28.448, 39.878) -> (28.194, 40.005)
  line L736 (28.194, 40.005) -> (28.067, 40.005)
  line L737 (28.067, 40.005) -> (27.94, 40.386)
  line L738 (27.94, 40.386) -> (28.194, 40.894)
  line L739 (28.194, 40.894) -> (27.94, 41.275)
  line L740 (27.94, 41.275) -> (27.559, 41.402)
  line L741 (27.559, 41.402) -> (27.178, 41.275)
  line L742 (27.178, 41.275) -> (27.051, 40.894)
  line L743 (27.051, 40.894) -> (27.178, 40.513)
  line L744 (27.178, 40.513) -> (27.305, 40.386)
  line L745 (27.305, 40.386) -> (27.051, 40.005)
  line L746 (26.6192, 39.9288) -> (26.8224, 39.9288)
  line L747 (28.3464, 39.9288) -> (28.4988, 39.9288)
  line L748 (26.5938, 40.0812) -> (27.1018, 40.0812)
  line L749 (28.0416, 40.0812) -> (28.5369, 40.0812)
  line L750 (26.6954, 40.2336) -> (27.2034, 40.2336)
  line L751 (27.9908, 40.2336) -> (28.4607, 40.2336)
  line L752 (26.797, 40.386) -> (27.305, 40.386)
  line L753 (27.94, 40.386) -> (28.448, 40.386)
  line L754 (26.6954, 40.5384) -> (27.1695, 40.5384)
  line L755 (28.0162, 40.5384) -> (28.448, 40.5384)
  line L756 (26.5938, 40.6908) -> (27.1187, 40.6908)
  line L757 (28.0924, 40.6908) -> (28.6004, 40.6908)
  line L758 (26.289, 40.8432) -> (27.0679, 40.8432)
  line L759 (28.1686, 40.8432) -> (28.8671, 40.8432)
  line L760 (26.289, 40.9956) -> (27.0849, 40.9956)
  line L761 (28.1263, 40.9956) -> (28.9433, 40.9956)
  line L762 (26.7123, 41.148) -> (27.1357, 41.148)
  line L763 (28.0247, 41.148) -> (28.5327, 41.148)
  line L764 (26.7631, 41.3004) -> (27.2542, 41.3004)
  line L765 (27.8638, 41.3004) -> (28.4819, 41.3004)
  line L766 (26.7631, 41.4528) -> (28.4649, 41.4528)
  line L767 (26.6615, 41.6052) -> (28.5157, 41.6052)
  line L768 (26.5599, 41.7576) -> (26.8986, 41.7576)
  line L769 (27.2034, 41.7576) -> (27.8892, 41.7576)
  line L770 (28.2956, 41.7576) -> (28.5665, 41.7576)
  line L771 (27.432, 41.91) -> (27.7707, 41.91)
  line L772 (27.432, 42.0624) -> (27.7199, 42.0624)
  line L773 (27.3812, 40.4622) -> (27.1272, 39.878)
  line L774 (27.1272, 39.878) -> (27.0002, 39.9542)
  line L775 (27.0002, 39.9542) -> (26.6954, 39.751)
  line L776 (26.6954, 39.751) -> (26.4668, 39.9796)
  line L777 (26.4668, 39.9796) -> (26.67, 40.3098)
  line L778 (26.67, 40.3098) -> (26.543, 40.64)
  line L779 (26.543, 40.64) -> (26.162, 40.7162)
  line L780 (26.162, 40.7162) -> (26.162, 41.0464)
  line L781 (26.162, 41.0464) -> (26.543, 41.0972)
  line L782 (26.543, 41.0972) -> (26.6954, 41.4274)
  line L783 (26.6954, 41.4274) -> (26.4668, 41.7576)
  line L784 (26.4668, 41.7576) -> (26.6954, 41.9862)
  line L785 (26.6954, 41.9862) -> (27.0256, 41.7576)
  line L786 (27.0256, 41.7576) -> (27.3304, 41.8846)
  line L787 (27.3304, 41.8846) -> (27.4066, 42.291)
  line L788 (27.4066, 42.291) -> (27.7368, 42.291)
  line L789 (27.7368, 42.291) -> (27.813, 41.8846)
  line L790 (27.813, 41.8846) -> (28.1178, 41.7576)
  line L791 (28.1178, 41.7576) -> (28.4734, 41.9862)
  line L792 (28.4734, 41.9862) -> (28.702, 41.7576)
  line L793 (28.702, 41.7576) -> (28.4734, 41.4274)
  line L794 (28.4734, 41.4274) -> (28.6004, 41.1226)
  line L795 (28.6004, 41.1226) -> (28.9814, 41.0464)
  line L796 (28.9814, 41.0464) -> (28.9814, 40.7162)
  line L797 (28.9814, 40.7162) -> (28.6258, 40.64)
  line L798 (28.6258, 40.64) -> (28.4734, 40.3098)
  line L799 (28.4734, 40.3098) -> (28.702, 39.9796)
  line L800 (28.702, 39.9796) -> (28.4734, 39.751)
  line L801 (28.4734, 39.751) -> (28.1686, 39.9542)
  line L802 (28.1686, 39.9542) -> (28.0162, 39.878)
  line L803 (28.0162, 39.878) -> (27.7876, 40.4622)
  arc A6 (27.7876, 40.4622) -> (27.3812, 40.4622) centre (27.5844, 40.8686) ccw
  line L804 (2.756, 25.719) -> (2.156, 25.719)
  line L805 (2.156, 25.719) -> (2.156, 24.919)
  line L806 (4.356, 25.719) -> (4.956, 25.719)
  line L807 (4.956, 25.719) -> (4.956, 24.919)
  line L808 (6.669, 26.519) -> (6.669, 23.519)
  line L809 (6.669, 23.519) -> (5.269, 23.519)
  line L810 (5.269, 23.519) -> (5.269, 26.519)
  line L811 (5.269, 26.519) -> (6.669, 26.519)
  line L812 (1.843, 26.519) -> (1.843, 23.519)
  line L813 (1.843, 23.519) -> (0.443, 23.519)
  line L814 (0.443, 23.519) -> (0.443, 26.519)
  line L815 (0.443, 26.519) -> (1.843, 26.519)
  line L816 (20.804, 29.399) -> (17.804, 29.399)
  line L817 (17.804, 29.399) -> (17.804, 30.799)
  line L818 (17.804, 30.799) -> (20.804, 30.799)
  line L819 (20.804, 30.799) -> (20.804, 29.399)
  line L820 (24.4, 33.7) -> (24.4, 30.7)
  line L821 (24.4, 30.7) -> (23, 30.7)
  line L822 (23, 30.7) -> (23, 33.7)
  line L823 (23, 33.7) -> (24.4, 33.7)
  line L824 (7.1635, 28.803) -> (5.6635, 28.803)
  line L825 (5.6635, 31.903) -> (7.1635, 31.903)
  line L826 (28.817, 21.691) -> (27.317, 21.691)
  line L827 (27.317, 24.791) -> (28.817, 24.791)
  line L828 (28.817, 29.184) -> (27.317, 29.184)
  line L829 (27.317, 32.284) -> (28.817, 32.284)
  line L830 (15.35, 32.35) -> (15.35, 30.85)
  line L831 (13.85, 30.85) -> (13.85, 32.35)
  line L832 (11.38, 9.483) -> (24.18, 9.483)
  line L833 (24.68, 9.983) -> (24.68, 22.783)
  line L834 (24.18, 23.283) -> (11.38, 23.283)
  line L835 (11.38, 23.283) -> (10.88, 22.783)
  line L836 (10.88, 22.783) -> (10.88, 9.983)
  line L837 (24.18, 23.283) -> (24.68, 22.783)
  line L838 (24.18, 9.483) -> (24.68, 9.983)
  line L839 (11.38, 9.483) -> (10.88, 9.983)
  circle A7 centre (11.88, 22.283) radius 0.5
  line L840 (20.575, 33.775) -> (15.225, 33.775)
  line L841 (15.225, 33.775) -> (15.225, 39.025)
  line L842 (15.225, 39.025) -> (20.575, 39.025)
  line L843 (20.575, 39.025) -> (20.575, 33.775)
  line L844 (13.203, 0.394) -> (9.403, 0.394)
  line L845 (9.403, 0.394) -> (9.403, 5.194)
  line L846 (9.403, 5.194) -> (13.203, 5.194)
  line L847 (13.203, 5.194) -> (13.203, 0.394)
  circle A8 centre (9.903, 4.694) radius 0.15
  line L848 (35.466, 20.943) -> (35.466, 32.943)
  line L849 (35.466, 32.943) -> (29.866, 32.943)
  line L850 (29.866, 32.943) -> (29.866, 20.943)
  line L851 (29.866, 20.943) -> (35.466, 20.943)
  line L852 (22.09, 0.0025) -> (31.25, 0.0025)
  line L853 (22.09, 0.0025) -> (22.09, 5.1575)
  line L854 (22.09, 5.1575) -> (31.25, 5.1575)
  line L855 (31.25, 5.1575) -> (31.25, 0.0025)
  line L856 (7.388, 17.402) -> (7.388, 16.202)
  line L857 (6.238, 15.152) -> (5.638, 15.152)
  line L858 (4.488, 16.202) -> (4.488, 17.402)
  line L859 (6.288, 18.402) -> (5.688, 18.402)
  circle A9 centre (4.519, 18.414) radius 0.1
  line L860 (26.678, 28.197) -> (26.678, 27.197)
  line L861 (26.678, 27.197) -> (27.678, 27.197)
  line L862 (27.678, 27.197) -> (27.678, 28.197)
  line L863 (27.678, 28.197) -> (26.678, 28.197)
  line L864 (26.678, 26.397) -> (26.678, 25.397)
  line L865 (26.678, 25.397) -> (27.678, 25.397)
  line L866 (27.678, 25.397) -> (27.678, 26.397)
  line L867 (27.678, 26.397) -> (26.678, 26.397)
  line L868 (16.01, 4.702) -> (16.01, 3.702)
  line L869 (16.01, 3.702) -> (17.01, 3.702)
  line L870 (17.01, 3.702) -> (17.01, 4.702)
  line L871 (17.01, 4.702) -> (16.01, 4.702)
  line L872 (16.01, 2.902) -> (16.01, 1.902)
  line L873 (16.01, 1.902) -> (17.01, 1.902)
  line L874 (17.01, 1.902) -> (17.01, 2.902)
  line L875 (17.01, 2.902) -> (16.01, 2.902)
  line L876 (6.723, 4.821) -> (5.723, 4.821)
  line L877 (5.723, 4.821) -> (5.723, 3.821)
  line L878 (5.723, 3.821) -> (6.723, 3.821)
  line L879 (6.723, 3.821) -> (6.723, 4.821)
  line L880 (6.723, 2.021) -> (5.723, 2.021)
  line L881 (5.723, 2.021) -> (5.723, 1.021)
  line L882 (5.723, 1.021) -> (6.723, 1.021)
  line L883 (6.723, 1.021) -> (6.723, 2.021)
  line L884 (7.755, 11.714) -> (7.755, 10.714)
  line L885 (7.755, 10.714) -> (8.755, 10.714)
  line L886 (8.755, 10.714) -> (8.755, 11.714)
  line L887 (8.755, 11.714) -> (7.755, 11.714)
  line L888 (7.755, 10.114) -> (7.755, 9.114)
  line L889 (7.755, 9.114) -> (8.755, 9.114)
  line L890 (8.755, 9.114) -> (8.755, 10.114)
  line L891 (8.755, 10.114) -> (7.755, 10.114)
  line L892 (6.104, 11.714) -> (6.104, 10.714)
  line L893 (6.104, 10.714) -> (7.104, 10.714)
  line L894 (7.104, 10.714) -> (7.104, 11.714)
  line L895 (7.104, 11.714) -> (6.104, 11.714)
  line L896 (6.104, 10.114) -> (6.104, 9.114)
  line L897 (6.104, 9.114) -> (7.104, 9.114)
  line L898 (7.104, 9.114) -> (7.104, 10.114)
  line L899 (7.104, 10.114) -> (6.104, 10.114)
  line L900 (10.66, 23.719) -> (10.66, 24.719)
  line L901 (10.66, 24.719) -> (9.66, 24.719)
  line L902 (9.66, 24.719) -> (9.66, 23.719)
  line L903 (9.66, 23.719) -> (10.66, 23.719)
  line L904 (10.66, 25.319) -> (10.66, 26.319)
  line L905 (10.66, 26.319) -> (9.66, 26.319)
  line L906 (9.66, 26.319) -> (9.66, 25.319)
  line L907 (9.66, 25.319) -> (10.66, 25.319)
  line L908 (13.365, 6.977) -> (12.365, 6.977)
  line L909 (12.365, 6.977) -> (12.365, 5.977)
  line L910 (12.365, 5.977) -> (13.365, 5.977)
  line L911 (13.365, 5.977) -> (13.365, 6.977)
  line L912 (11.765, 6.977) -> (10.765, 6.977)
  line L913 (10.765, 6.977) -> (10.765, 5.977)
  line L914 (10.765, 5.977) -> (11.765, 5.977)
  line L915 (11.765, 5.977) -> (11.765, 6.977)
  line L916 (25.027, 9.047) -> (25.027, 8.047)
  line L917 (25.027, 8.047) -> (26.027, 8.047)
  line L918 (26.027, 8.047) -> (26.027, 9.047)
  line L919 (26.027, 9.047) -> (25.027, 9.047)
  line L920 (25.027, 7.447) -> (25.027, 6.447)
  line L921 (25.027, 6.447) -> (26.027, 6.447)
  line L922 (26.027, 6.447) -> (26.027, 7.447)
  line L923 (26.027, 7.447) -> (25.027, 7.447)
  line L924 (26.027, 23.719) -> (26.027, 24.719)
  line L925 (26.027, 24.719) -> (25.027, 24.719)
  line L926 (25.027, 24.719) -> (25.027, 23.719)
  line L927 (25.027, 23.719) -> (26.027, 23.719)
  line L928 (26.027, 25.319) -> (26.027, 26.319)
  line L929 (26.027, 26.319) -> (25.027, 26.319)
  line L930 (25.027, 26.319) -> (25.027, 25.319)
  line L931 (25.027, 25.319) -> (26.027, 25.319)
  line L932 (28.329, 28.097) -> (28.329, 27.097)
  line L933 (28.329, 27.097) -> (29.329, 27.097)
  line L934 (29.329, 27.097) -> (29.329, 28.097)
  line L935 (29.329, 28.097) -> (28.329, 28.097)
  line L936 (28.329, 26.497) -> (28.329, 25.497)
  line L937 (28.329, 25.497) -> (29.329, 25.497)
  line L938 (29.329, 25.497) -> (29.329, 26.497)
  line L939 (29.329, 26.497) -> (28.329, 26.497)
  line L940 (7.628, 23.373) -> (8.628, 23.373)
  line L941 (8.628, 23.373) -> (8.628, 24.373)
  line L942 (8.628, 24.373) -> (7.628, 24.373)
  line L943 (7.628, 24.373) -> (7.628, 23.373)
  line L944 (7.628, 26.173) -> (8.628, 26.173)
  line L945 (8.628, 26.173) -> (8.628, 27.173)
  line L946 (8.628, 27.173) -> (7.628, 27.173)
  line L947 (7.628, 27.173) -> (7.628, 26.173)
  line L948 (20.071, 41.267) -> (20.071, 40.267)
  line L949 (20.071, 40.267) -> (21.071, 40.267)
  line L950 (21.071, 40.267) -> (21.071, 41.267)
  line L951 (21.071, 41.267) -> (20.071, 41.267)
  line L952 (22.871, 41.267) -> (22.871, 40.267)
  line L953 (22.871, 40.267) -> (23.871, 40.267)
  line L954 (23.871, 40.267) -> (23.871, 41.267)
  line L955 (23.871, 41.267) -> (22.871, 41.267)
  line L956 (8.755, 18.512) -> (8.755, 19.512)
  line L957 (8.755, 19.512) -> (7.755, 19.512)
  line L958 (7.755, 19.512) -> (7.755, 18.512)
  line L959 (7.755, 18.512) -> (8.755, 18.512)
  line L960 (8.755, 20.112) -> (8.755, 21.112)
  line L961 (8.755, 21.112) -> (7.755, 21.112)
  line L962 (7.755, 21.112) -> (7.755, 20.112)
  line L963 (7.755, 20.112) -> (8.755, 20.112)
  line L964 (18.973, 41) -> (17.973, 41)
  line L965 (17.973, 41) -> (17.973, 40)
  line L966 (17.973, 40) -> (18.973, 40)
  line L967 (18.973, 40) -> (18.973, 41)
  line L968 (17.373, 41) -> (16.373, 41)
  line L969 (16.373, 41) -> (16.373, 40)
  line L970 (16.373, 40) -> (17.373, 40)
  line L971 (17.373, 40) -> (17.373, 41)
  line L972 (21.5, 37.2) -> (21.5, 36.2)
  line L973 (21.5, 36.2) -> (22.5, 36.2)
  line L974 (22.5, 36.2) -> (22.5, 37.2)
  line L975 (22.5, 37.2) -> (21.5, 37.2)
  line L976 (21.5, 35.6) -> (21.5, 34.6)
  line L977 (21.5, 34.6) -> (22.5, 34.6)
  line L978 (22.5, 34.6) -> (22.5, 35.6)
  line L979 (22.5, 35.6) -> (21.5, 35.6)
  line L980 (20.6, 32.6) -> (19.6, 32.6)
  line L981 (19.6, 32.6) -> (19.6, 31.6)
  line L982 (19.6, 31.6) -> (20.6, 31.6)
  line L983 (20.6, 31.6) -> (20.6, 32.6)
  line L984 (19, 32.6) -> (18, 32.6)
  line L985 (18, 32.6) -> (18, 31.6)
  line L986 (18, 31.6) -> (19, 31.6)
  line L987 (19, 31.6) -> (19, 32.6)
  line L988 (21.5, 33.5) -> (21.5, 32.5)
  line L989 (21.5, 32.5) -> (22.5, 32.5)
  line L990 (22.5, 32.5) -> (22.5, 33.5)
  line L991 (22.5, 33.5) -> (21.5, 33.5)
  line L992 (21.5, 31.9) -> (21.5, 30.9)
  line L993 (21.5, 30.9) -> (22.5, 30.9)
  line L994 (22.5, 30.9) -> (22.5, 31.9)
  line L995 (22.5, 31.9) -> (21.5, 31.9)
  line L996 (13.2, 38.9) -> (13.2, 37.9)
  line L997 (13.2, 37.9) -> (14.2, 37.9)
  line L998 (14.2, 37.9) -> (14.2, 38.9)
  line L999 (14.2, 38.9) -> (13.2, 38.9)
  line L1000 (13.2, 37.3) -> (13.2, 36.3)
  line L1001 (13.2, 36.3) -> (14.2, 36.3)
  line L1002 (14.2, 36.3) -> (14.2, 37.3)
  line L1003 (14.2, 37.3) -> (13.2, 37.3)
  line L1004 (11.5, 39) -> (11.5, 38)
  line L1005 (11.5, 38) -> (12.5, 38)
  line L1006 (12.5, 38) -> (12.5, 39)